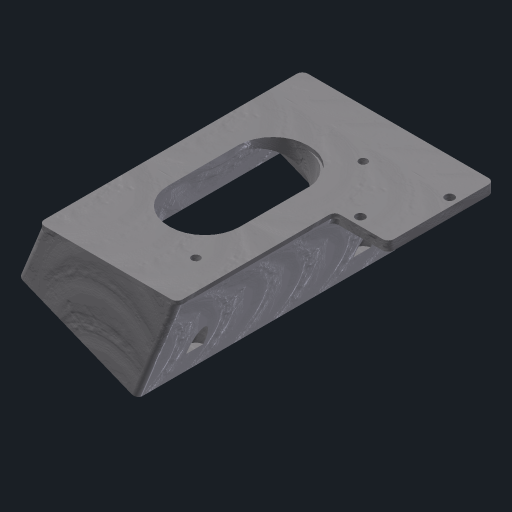
# Autodesk Inventor part: SOPORTE_CAMARA_2
Saved by Autodesk Inventor 2024.3 (Build 283343000, 343)
## iProperties
Created: 2024-07-21
Part Number: SOPORTE_CAMARA_2
Material: Steel, Mild, Welded
Document SubType Name: Modeling
Designer: Niler
Density: 7.85 g/cm^3
Appearance: Weld - Steel Mild
Author: Niler
Autodesk Inventor part; units mm, degrees
ref_plane "YZ Plane" through (0, 0, 0) normal (1, 0, 0) x (0, 1, 0)
ref_plane "XZ Plane" through (0, 0, 0) normal (0, 1, 0) x (-1, 0, 0)
ref_plane "XY Plane" through (0, 0, 0) normal (0, 0, 1) x (1, 0, 0)
sketch "Sketch1" plane through (0, 0, 0) normal (0, 1, 0) x (-1, 0, 0)
  line L0 (-17.5, 40) -> (17.5, 40)
  line L1 (17.5, 40) -> (17.5, -40)
  line L2 (17.5, -40) -> (-17.5, -40)
  line L3 (-17.5, -40) -> (-17.5, 40)
  line L4 (-17.5, 40) -> (17.5, -40) construction
  line L5 (17.5, 40) -> (-17.5, -40) construction
  line L6 (17.8, -40.3) -> (17.8, 40.3)
  line L7 (17.8, 40.3) -> (-17.8, 40.3)
  line L8 (-17.8, 40.3) -> (-17.8, -40.3)
  line L9 (-17.8, -40.3) -> (17.8, -40.3)
  line L10 (24.8, 47.3) -> (24.8, -47.3)
  line L11 (24.8, -47.3) -> (-24.8, -47.3)
  line L12 (-24.8, -47.3) -> (-24.8, 47.3)
  line L13 (-24.8, 47.3) -> (24.8, 47.3)
  line L14 (0, 12.5) -> (0, -12.5) construction
  line L15 (-12.5, 12.5) -> (-12.5, -12.5)
  line L16 (12.5, -12.5) -> (12.5, 12.5)
  arc A0 (12.5, 12.5) -> (-12.5, 12.5) centre (0, 12.5) ccw
  arc A1 (-12.5, -12.5) -> (12.5, -12.5) centre (0, -12.5) ccw
  point P0 (0, 0)
  dimension "d0" = 35
  dimension "d1" = 80
  dimension "d2" = 0.3
  dimension "d3" = 7
  dimension "d4" = 25
  dimension "d5" = 25
  constraints: 36 end point, 7 parallel, 4 point on circle, 4 tangent, 3 midpoint, 3 perpendicular, 2 centre point, 1 horizontal, 1 vertical, 6 other
  measures "d0" distance of L1.end L2.end
  measures "d1" distance of L0.end L1.end
  measures "d2" distance between parallel lines of L1 L6
  measures "d3" distance between parallel lines of L6 L10
  measures "d4" diameter of A1
  measures "d5" distance of L14.start L14.end
extrude "Extrusion1" add sketch "Sketch1" along normal blind 3 contours L0 L1 L2 L3 | L9 L8 L7 L6 | L10 L11 L12 L13
sketch "Sketch2" plane through (-24.8, 0, 47.3) normal (0, 0, 1) x (1, 0, 0)
  line L0 (0, 0) -> (49.6, 0)
  line L1 (49.6, 0) -> (49.6, 3)
  line L2 (0, 3) -> (49.6, 3)
  line L3 (0, 0) -> (0, 3)
  line L4 (49.6, 0) -> (42.639627, -17.227528)
  line L5 (42.639627, -17.227528) -> (0, 0)
  point P0 (24.8, 0)
  dimension "d8" = 68
  constraints: 4 end point, 1 perpendicular
  measures "d8" angle of L0 L4
extrude "Extrusion2" add sketch "Sketch2" against normal up to surface (94.6 mm away) contours L0 L4 L5
sketch "Sketch3" plane through (-24.8, 0, -47.3) normal (-0.3746066, -0.9271839, 0) x (0.9271839, -0.3746066, 0)
  line L0 (44.864499, 94.6) -> (44.864499, 0)
  line L1 (44.864499, 0) -> (-1.12382, 0)
  line L2 (-1.12382, 0) -> (-1.12382, 94.6)
  line L3 (-1.12382, 94.6) -> (44.864499, 94.6)
  ellipse E0 centre (21.87034, 59.8) end of major axis (21.87034, 72.3) minor radius 11.589798 (33.460138, 59.8) -> (10.280542, 59.8) ccw
  line L4 (10.280542, 59.8) -> (10.280542, 34.8)
  ellipse E1 centre (21.87034, 34.8) end of major axis (21.87034, 22.3) minor radius 11.589798 (10.280542, 34.8) -> (33.460138, 34.8) ccw
  line L5 (33.460138, 34.8) -> (33.460138, 59.8)
  point P0 (22.99416, 47.3)
  constraints: 2 other
extrude "Extrusion3" cut sketch "Sketch3" against normal through all contours L5 E1 L4 E0
sketch "Sketch4" plane through (-24.8, 0, -47.3) normal (-0.3746066, -0.9271839, 0) x (0.9271839, -0.3746066, 0)
  ellipse E0 centre (21.87034, 34.8) end of major axis (21.87034, 22.3) minor radius 11.589798 (10.280542, 34.8) -> (33.460138, 34.8) ccw
  line L0 (10.280542, 34.8) -> (10.280542, 59.8)
  ellipse E1 centre (21.87034, 59.8) end of major axis (21.87034, 72.3) minor radius 11.589798 (33.460138, 59.8) -> (10.280542, 59.8) ccw
  line L1 (33.460138, 59.8) -> (33.460138, 34.8)
  line L2 (0, 0) -> (45.988319, 0)
  line L3 (45.988319, 94.6) -> (45.988319, 0)
  line L4 (0, 94.6) -> (45.988319, 94.6)
  line L5 (0, 0) -> (0, 94.6)
  line L6 (7, 87.6) -> (38.988319, 87.6)
  line L7 (38.988319, 87.6) -> (38.988319, 7)
  line L8 (38.988319, 7) -> (7, 7)
  line L9 (7, 7) -> (7, 87.6)
  point P0 (22.99416, 47.3)
  dimension "d13" = 7
  constraints: 8 end point, 5 other
  measures "d13" distance between parallel lines of L5 L9
extrude "Extrusion4" add sketch "Sketch4" along normal blind 20 contours L5 L4 L3 L2
sketch "Sketch5" plane through (-18.309713, -2.622246, -40.3) normal (-0.3746066, -0.9271839, 0) x (0.9271839, -0.3746066, 0)
  line L0 (0, 80.6) -> (0, 0)
  line L1 (0, 0) -> (31.988319, 0)
  line L2 (31.988319, 0) -> (31.988319, 80.6)
  line L3 (31.988319, 80.6) -> (0, 80.6)
  ellipse E0 centre (14.87034, 27.8) end of major axis (14.87034, 15.3) minor radius 11.589798 (3.280542, 27.8) -> (26.460138, 27.8) ccw
  line L4 (3.280542, 27.8) -> (3.280542, 52.8)
  ellipse E1 centre (14.87034, 52.8) end of major axis (14.87034, 65.3) minor radius 11.589798 (26.460138, 52.8) -> (3.280542, 52.8) ccw
  line L5 (26.460138, 52.8) -> (26.460138, 27.8)
  point P0 (15.99416, 40.3)
  constraints: 2 other
extrude "Extrusion5" cut sketch "Sketch5" against normal blind 2
sketch "Sketch8" plane through (0, 3, 0) normal (0, 1, 0) x (1, 0, 0)
  line L0 (24.8, -47.3) -> (24.8, 47.3) projected
  line L1 (24.8, 47.3) -> (-24.8, 47.3) projected
  line L2 (-24.8, 47.3) -> (-24.8, -47.3) projected
  line L3 (-24.8, -47.3) -> (24.8, -47.3) projected
  arc A0 (0, -25) -> (12.5, -12.5) centre (0, -12.5) ccw projected
  arc A1 (-12.5, -12.5) -> (0, -25) centre (0, -12.5) ccw projected
  line L4 (-12.5, -12.5) -> (-12.5, 12.5) projected
  arc A2 (0, 25) -> (-12.5, 12.5) centre (0, 12.5) ccw projected
  arc A3 (12.5, 12.5) -> (0, 25) centre (0, 12.5) ccw projected
  line L5 (12.5, 12.5) -> (12.5, -12.5) projected
  circle A4 centre (14.3, -30) radius 1.5
  circle A5 centre (14.3, 30) radius 1.5
  line L6 (14.3, -30) -> (14.3, 30) construction
  circle A6 centre (14.3, -30) radius 3.1
  circle A7 centre (14.3, 30) radius 3.1
  point P0 (0, 0)
  point P1 (14.3, 0)
  dimension "d31" = 3
  dimension "d32" = 60
  dimension "d35" = 10.5
  dimension "d36" = 6.2
  constraints: 4 centre point, 2 coincident, 2 end point, 2 equal radius, 1 horizontal alignment, 1 midpoint, 1 vertical, 1 vertical alignment
  measures "d31" diameter of A5
  measures "d32" distance of L6.end L6.start
  measures "d35" distance from line of L0 L6.start
  measures "d36" diameter of A6
extrude "Extrusion8" cut sketch "Sketch8" against normal blind 30 contours A4 | A5 | A6 | A7
extrude "Extrusion9" add sketch "Sketch8" against normal blind 5 contours A6 | A7
sketch "Sketch10" plane through (24.8, 3, -47.3) normal (0, 0, -1) x (-1, 0, 0)
  line L0 (49.6, -3) -> (49.6, 0)
  line L1 (0, 0) -> (49.6, 0)
  line L2 (0, -3) -> (0, 0)
  line L3 (0, -3) -> (14.452505, -38.771205)
  line L4 (57.092132, -21.543677) -> (14.452505, -38.771205)
  line L5 (49.6, -3) -> (57.092132, -21.543677)
  line L6 (0.808052, -5) -> (-19.191948, -5)
  line L7 (-19.191948, -5) -> (-19.191948, 0)
  line L8 (-19.191948, 0) -> (0, 0)
  point P0 (24.8, -3)
  dimension "d40" = 20
  dimension "d41" = 5
  constraints: 6 end point, 1 horizontal, 1 perpendicular, 1 point on line, 1 vertical
  measures "d40" distance of L6.start L6.end
  measures "d41" distance between parallel lines of L6 L8
extrude "Extrusion10" add sketch "Sketch10" against normal blind 38 contours L2 L3 L6 L7 L8
sketch "Sketch11" plane through (23.991948, -2, -47.3) normal (0, -1, 0) x (1, 0, 0)
  line L0 (20, 0) -> (0, 0)
  line L1 (20, 0) -> (20, 38)
  line L2 (0, 0) -> (0, 38)
  line L3 (20, 38) -> (0.808052, 38)
  line L4 (20, 0) -> (4, 0)
  line L5 (4, 0) -> (4, 38)
  line L6 (4, 38) -> (20, 38)
  line L7 (20, 38) -> (20, 0)
  line L8 (18, 10) -> (17, 10) construction
  line L9 (17, 10) -> (17, 13) construction
  line L10 (17, 13) -> (20, 13) construction
  line L11 (20, 13) -> (20, 0) construction
  line L12 (4, 38) -> (7, 38) construction
  line L13 (7, 38) -> (7, 35) construction
  line L14 (7, 35) -> (4, 35) construction
  line L15 (4, 35) -> (4, 38) construction
  circle A0 centre (17, 13) radius 1.65
  circle A1 centre (7, 35) radius 1.65
  point P0 (-23.991948, 47.3)
  dimension "d44" = 16
  dimension "d45" = 3
  dimension "d46" = 3
  dimension "d47" = 3
  dimension "d48" = 3
  dimension "d49" = 3.3
  dimension "d50" = 3.3
  dimension "d60" = 28
  constraints: 24 end point, 6 parallel, 3 horizontal, 3 perpendicular, 2 centre point, 2 coincident, 1 point on line
  measures "d44" distance between parallel lines of L1 L5
  measures "d45" distance of L9.end L10.end
  measures "d46" distance of L8.end L9.end
  measures "d47" distance of L13.end L14.end
  measures "d48" distance of L12.end L13.end
  measures "d49" diameter of A0
  measures "d50" diameter of A1
  measures "d60" distance between parallel lines of L8 L3
extrude "Extrusion11" cut sketch "Sketch11" against normal through all contours A0 | A1
fillet "Fillet1" radius 2 4 edges at (43.9919, 0.5, -47.3) (43.9919, 0.5, -9.3) (24.8, 1.5, -9.3) (24.396, -1, -9.3)
sketch "Sketch12" plane through (-32.292132, -18.543677, -47.3) normal (-0.3746066, -0.9271839, 0) x (0.9271839, -0.3746066, 0)
  line L0 (0, 0) -> (45.988319, 0)
  line L1 (45.988319, 0) -> (45.988319, 94.6)
  line L2 (45.988319, 94.6) -> (0, 94.6)
  line L3 (0, 94.6) -> (0, 0)
  line L4 (7, 87.6) -> (38.988319, 87.6)
  line L5 (38.988319, 87.6) -> (38.988319, 7)
  line L6 (38.988319, 7) -> (7, 7)
  line L7 (7, 7) -> (7, 87.6)
  line L8 (0, 0) -> (7, 0)
  line L9 (7, 0) -> (7, 7)
  line L10 (7, 7) -> (0, 7)
  line L11 (0, 7) -> (0, 0)
  circle A0 centre (3.5, 3.5) radius 1.5
  line L12 (22.99416, 47.3) -> (15.368168, 47.3)
  line L13 (15.368168, 47.3) -> (22.99416, 47.3)
  line L14 (22.99416, 47.3) -> (22.99416, 38.83375)
  circle A1 centre (3.5, 91.1) radius 1.5
  circle A2 centre (42.488319, 3.5) radius 1.5
  circle A3 centre (42.488319, 91.1) radius 1.5
  point P0 (0, 3.5)
  point P1 (3.5, 7)
  dimension "d55" = 3
  constraints: 14 end point, 4 centre point, 3 equal length, 3 symmetric about line, 2 horizontal, 2 midpoint, 1 horizontal alignment, 1 perpendicular, 1 vertical, 1 vertical alignment, 3 other
  measures "d55" diameter of A0
extrude "Extrusion12" cut sketch "Sketch12" against normal blind 15 contours A0 | A1 | A2 | A3
fillet "Fillet2" radius 2 7 edges at (17.1697, -18.8856, -47.3) (-28.5461, -9.2718, -47.3) (-24.8, 1.5, -47.3) (-24.8, 1.5, 47.3) (-28.5461, -9.2718, 47.3) (17.5737, -17.8856, 47.3) (24.8, 1.5, 47.3)
fillet "Fillet3" radius 3 3 edges at (-24.2142, -0.1139, 46.7142) (-24.2142, -0.1139, -46.7142) (-24.8, 0, 0)
sketch "Sketch13" plane through (0, 3, 0) normal (0, 1, 0) x (1, 0, 0)
  line L0 (-52.220504, -87.222351) -> (50.526866, -87.222351)
  line L1 (50.526866, -87.222351) -> (50.526866, 68.404152)
  line L2 (50.526866, 68.404152) -> (-52.220504, 68.404152)
  line L3 (-52.220504, 68.404152) -> (-52.220504, -87.222351)
  point P0 (0, 0)
  constraints: 8 end point, 2 parallel, 1 horizontal, 1 perpendicular
extrude "Extrusion13" cut sketch "Sketch13" against normal blind 1.5
body "Solid1"
